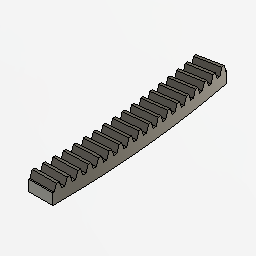
Rack_Curved (Autodesk Fusion 360 design; units mm, degrees)
Autodesk Fusion 360 part; units mm, degrees
note: some values were not read from the file. Chosen so that the rebuilt part matches the saved one: which face or edge a step refers to. Set by a fixed rule: which sketch regions a step uses.
sketch "Curve Base Shape" plane through (0, 0, 0) normal (0, 0, 1) x (1, 0, 0) in component "Rack Curved"
  arc A0 (0, 0) -> (-6.0719, 61.6485) centre (-316, 0) ccw construction
  line L0 (-4, 0) -> (4, 0) construction
  line L1 (-9.995, 60.8682) -> (-2.1487, 62.4289) construction
  arc A1 (-4, 0) -> (-9.995, 60.8682) centre (-316, 0) ccw construction
  arc A2 (4, 0) -> (-2.1487, 62.4289) centre (-316, 0) ccw construction
  line L2 (-5.5024, 30.5813) -> (2.4591, 31.3655) construction
  dimension "d104" = 11.25
  dimension "d109" = 4
  dimension "d110" = 4
  dimension "d111" = 316
  measures "d104" angle of L0 L1
  measures "d109" distance of A0 A2
  measures "d110" distance of A0 A1
  measures "d111" radius of A0
sketch "Curve Base" plane through (0, 0, 0) normal (0, 0, 1) x (1, 0, 0) in component "Rack Curved"
  arc A0 (-4, 0) -> (-9.995, 60.8682) centre (-316, 0) ccw construction
  line L0 (-4, 0) -> (4, 0) construction
  arc A1 (4, 0) -> (-2.1487, 62.4289) centre (-316, 0) ccw construction
  line L1 (-9.995, 60.8682) -> (-2.1487, 62.4289) construction
  line L2 (-5.5024, 30.5813) -> (2.4591, 31.3655) construction
  arc A2 (3.9, 0.1) -> (-2.2273, 62.3113) centre (-316, 0) ccw
  arc A3 (-3.9, 0.1) -> (-9.8774, 60.7896) centre (-316, 0) ccw
  line L3 (-9.8774, 60.7896) -> (-2.2273, 62.3113)
  line L4 (-3.9, 0.1) -> (3.9, 0.1)
  circle A4 centre (0, 4) radius 2.475 construction
  line L5 (0, 1.525) -> (0, 4) construction
  circle A5 centre (-1.9137, 34.9542) radius 2.475 construction
  line L6 (-1.9137, 34.9542) -> (-1.5216, 30.9734) construction
  circle A6 centre (-1.5216, 30.9734) radius 1.525
  circle A7 centre (-0.1013, 8) radius 1.5263
  arc A8 (0, 0) -> (-6.0719, 61.6485) centre (-316, 0) ccw
  arc A9 (-2.4534, 1.525) -> (-3.9595, 30.7333) centre (-316, 0) ccw
  arc A10 (2.4967, 1.525) -> (0.9666, 31.2185) centre (-316, 0) ccw
  line L7 (-2.4534, 1.525) -> (2.4967, 1.525)
  arc A11 (-3.9595, 30.7333) -> (-8.1806, 59.6742) centre (-316, 0) ccw
  line L8 (-8.1806, 59.6742) -> (-3.3256, 60.6399)
  arc A12 (0.9666, 31.2185) -> (-3.3256, 60.6399) centre (-316, 0) ccw
  circle A13 centre (-4.6105, 53.7825) radius 1.5263
  dimension "d112" = 0.1
  dimension "d114" = 0.1
  dimension "d115" = 0.1
  dimension "d116" = 0.1
  dimension "d117" = 4
  dimension "d118" = 4.95
  dimension "d120" = 4.95
  dimension "d121" = 4
  dimension "d160" = 8
  measures "d112" distance of L1 L3
  measures "d114" distance of A1 A2
  measures "d115" distance of A0 A3
  measures "d116" distance of L0 L4
  measures "d117" distance of L0 A4.centre
  measures "d118" diameter of A4
  measures "d120" diameter of A5
  measures "d121" distance of L2 A5.centre
  measures "d160" distance of L0 A7.centre
sketch "Section" plane through (0, 0, 0) normal (0, 1, 0) x (1, 0, 0) in component "Rack Curved"
  line L0 (-4, -5.9) -> (4, -5.9)
  line L1 (4, -5.9) -> (4, 0)
  line L2 (-4, 0) -> (-4, -5.9)
  line L3 (0, 0) -> (0, -5.9) construction
  line L4 (-316, -5.9) -> (-316, 0) construction
  line L5 (-4, -3.2) -> (4, -3.2)
  line L6 (0, -2.3) -> (2.4591, -2.3) construction
  line L7 (2.4591, -2.3) -> (2.4591, 0) construction
  line L8 (-4, 0) -> (4, 0)
  line L9 (4, -3.8) -> (-4, -3.8) construction
  point P0 (-4, -1.8)
  point P1 (2.4591, 0)
  dimension "d74" = 5.9
  dimension "d76" = 316
  dimension "d99" = 4
  dimension "d101" = 0.9
  dimension "d124" = 3.2
  dimension "d161" = 3.8
  measures "d74" distance of L0.end L1.end
  measures "d76" distance of L3.start L4.end
  measures "d99" distance of L3 P0
  measures "d101" distance of L5 L6
  measures "d124" distance of L5.end L8
  measures "d161" distance of L8 L9.end
sketch "Tooth" plane through (0, 0, 0) normal (1, 0, 0) x (0, 1, 0) in component "Rack Curved"
  line L0 (0, 0) -> (0, 5.9) construction
  line L1 (0, 5.9) -> (1.2882, 5.9)
  line L2 (1.2882, 5.9) -> (0.5239, 3.8)
  line L3 (0.5239, 3.8) -> (0, 3.8)
  line L4 (0, 4.85) -> (0.9061, 4.85) construction
  line L5 (0, 5.9) -> (-1.2882, 5.9)
  line L6 (-1.2882, 5.9) -> (-0.5239, 3.8)
  line L7 (-0.5239, 3.8) -> (0, 3.8)
  dimension "d87" = 3.8
  dimension "d88" = 20
  dimension "d89" = 0.9061
  measures "d87" distance of L0.start L3
  measures "d88" angle of L0 L2
  measures "d89" distance of L4.start L4.end
extrude "Extrude2" add sketch "Curve Base" along normal up to surface (5.9 mm away) in component "Rack Curved"
extrude "Extrude4" cut sketch "Curve Base" along normal up to surface (2.3 mm away) contours A6 A7 A8 A9 L7 A11 L8 A13 | A6 A7 A8 A10 L7 L8 A12 A13 | A6 A8 | A6 A8 in component "Rack Curved"
chamfer "Chamfer2" distance 0.3 angle 45 10 edges at (-5.4028, 30.5911, 0) (-6.0524, 61.5505, 0) (2.3596, 31.3557, 0) (0, 0.1, 0) (0.9666, 31.2185, 0) (-1.5243, 8.5519, 0) (-3.9595, 30.7333, 0) (0.0216, 1.525, 0) (-5.7531, 60.1571, 0) (-6.0335, 54.3344, 0) in component "Rack Curved"
extrude "Extrude5" add sketch "Curve Base" along normal up to surface (2.3 mm away) contours A6 A8 | A6 A8 in component "Rack Curved"
chamfer "Chamfer1" distance 0.3 angle 45 1 edges at (-2.9434, 30.422, 0) in component "Rack Curved"
pattern_circular "C-Pattern2" count 3 over 5.625 about axis through (-316, 0, 0) along (0, 0, 1) both ways of "Extrude5", "Chamfer1" in component "Rack Curved"
extrude "Extrude3" cut sketch "Tooth" against normal through all and the other way through all in component "Rack Curved"
pattern_circular "C-Pattern1" count 19 over 11.25 about axis through (-316, 0, 0) along (0, 0, 1) of "Extrude3" in component "Rack Curved"
component "Rack Curved" placed x (1, 0, 0) y (0, 1, 0) z (0, 0, 1) at (0, 0, 0)
equation "DeltaX = 8 mm"
equation "DeltaY = 8 mm"
equation "DeltaZ = 3.2 mm"
equation "Wall = 0.8 mm"
equation "Gap = 0.1 mm"
equation "KnobDiameter = 4.95 mm"
equation "KnobHeight = 1.8 mm"
equation "WallZ = 1 mm"
equation "BasePlateChamfer = 0.3 mm"
equation "CurveCenterRadius = 39.5" comment "38.5 / 39.5 / 40.5 / 41.5"
equation "CurveAngle = ( 90 / 8 ) * 1 deg"
equation "Height = 5.9 mm"
equation "BaseHeight = 3.8 mm"
equation "d74 = Height"
equation "d76 = CurveCenterRadius * DeltaX"
equation "Module = 1 mm"
equation "CurveLength = ( PI * CurveAngle / 180 deg ) * DeltaX * ( CurveCenterRadius - 0.5 )"
equation "NumTeeth = floor(CurveLength / ( PI * Module ))"
equation "PressureAngle = 20 deg"
equation "d87 = BaseHeight"
equation "d88 = PressureAngle"
equation "d89 = CurveLength / NumTeeth / 4 + Gap"
equation "d92 = NumTeeth"
equation "d93 = CurveAngle"
equation "d99 = DeltaX / 2"
equation "d101 = ( 6 * 0.15 ) * 1 mm"
equation "d104 = CurveAngle"
equation "d109 = DeltaX / 2"
equation "d110 = DeltaX / 2"
equation "d111 = CurveCenterRadius * DeltaX"
equation "d112 = Gap"
equation "d114 = Gap"
equation "d115 = Gap"
equation "d116 = Gap"
equation "d117 = DeltaY / 2"
equation "d118 = KnobDiameter"
equation "d120 = KnobDiameter"
equation "d121 = DeltaY / 2"
equation "d124 = DeltaZ"
equation "d135 = CurveAngle / 2"
equation "d136 = BasePlateChamfer"
equation "d137 = BasePlateChamfer"
equation "d160 = DeltaY"
equation "d161 = BaseHeight"
named bodies: "Rack Curved"
